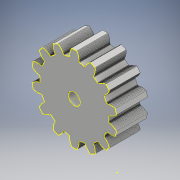
# Autodesk Inventor part: Engranaje_V_G
Saved by Autodesk Inventor 2017 (Build 210142000, 142)
## iProperties
Created: 2016-10-02
Part Number: Engranaje_V_G
Material: Generic
Document SubType Name: Modeling
Designer: CASA
Density: 1 g/cm^3
Appearance: Default
Author: CASA
Autodesk Inventor part; units mm, degrees
(part 1 of 2)
ref_plane "YZ Plane" through (0, 0, 0) normal (1, 0, 0) x (0, 1, 0)
ref_plane "XZ Plane" through (0, 0, 0) normal (0, 1, 0) x (-1, 0, 0)
ref_plane "XY Plane" through (0, 0, 0) normal (0, 0, 1) x (1, 0, 0)
sketch "Sketch4" plane through (0, 0, 0) normal (0, 1, 0) x (-1, 0, 0)
  line L0 (0.4842, 0.4117) -> (0.4817, 0.3929)
  line L1 (0.4817, 0.3929) -> (0.4745, 0.3754)
  line L2 (0.4745, 0.3754) -> (0.4629, 0.3604)
  line L3 (0.4629, 0.3604) -> (0.4479, 0.3489)
  line L4 (0.4479, 0.3489) -> (0.4304, 0.3416)
  line L5 (0.4304, 0.3416) -> (0.4117, 0.3392)
  line L6 (0.4117, 0.3392) -> (0.3929, 0.3416)
  line L7 (0.3929, 0.3416) -> (0.3754, 0.3489)
  line L8 (0.3754, 0.3489) -> (0.3604, 0.3604)
  line L9 (0.3604, 0.3604) -> (0.3489, 0.3754)
  line L10 (0.3489, 0.3754) -> (0.3416, 0.3929)
  line L11 (0.3416, 0.3929) -> (0.3392, 0.4117)
  line L12 (0.3392, 0.4117) -> (0.3416, 0.4304)
  line L13 (0.3416, 0.4304) -> (0.3489, 0.4479)
  line L14 (0.3489, 0.4479) -> (0.3604, 0.4629)
  line L15 (0.3604, 0.4629) -> (0.3754, 0.4745)
  line L16 (0.3754, 0.4745) -> (0.3929, 0.4817)
  line L17 (0.3929, 0.4817) -> (0.4117, 0.4842)
  line L18 (0.4117, 0.4842) -> (0.4304, 0.4817)
  line L19 (0.4304, 0.4817) -> (0.4479, 0.4745)
  line L20 (0.4479, 0.4745) -> (0.4629, 0.4629)
  line L21 (0.4629, 0.4629) -> (0.4745, 0.4479)
  line L22 (0.4745, 0.4479) -> (0.4817, 0.4304)
  line L23 (0.4817, 0.4304) -> (0.4842, 0.4117)
  line L24 (0.0797, 0.4378) -> (0.0785, 0.4393)
  line L25 (0.0785, 0.4393) -> (0.0772, 0.4404)
  line L26 (0.0772, 0.4404) -> (0.076, 0.4413)
  line L27 (0.076, 0.4413) -> (0.0747, 0.442)
  line L28 (0.0747, 0.442) -> (0.0734, 0.4426)
  line L29 (0.0734, 0.4426) -> (0.0708, 0.4437)
  line L30 (0.0708, 0.4437) -> (0.0682, 0.4445)
  line L31 (0.0682, 0.4445) -> (0.0656, 0.4451)
  line L32 (0.0656, 0.4451) -> (0.0604, 0.4462)
  line L33 (0.0604, 0.4462) -> (0.0552, 0.4478)
  line L34 (0.0552, 0.4478) -> (0.05, 0.4497)
  line L35 (0.05, 0.4497) -> (0.0449, 0.452)
  line L36 (0.0449, 0.452) -> (0.0398, 0.4545)
  line L37 (0.0398, 0.4545) -> (0.0348, 0.4573)
  line L38 (0.0348, 0.4573) -> (0.0298, 0.4603)
  line L39 (0.0298, 0.4603) -> (0.0248, 0.4636)
  line L40 (0.0248, 0.4636) -> (0.0199, 0.467)
  line L41 (0.0199, 0.467) -> (0.015, 0.4707)
  line L42 (0.015, 0.4707) -> (0.0102, 0.4745)
  line L43 (0.0102, 0.4745) -> (0.0055, 0.4786)
  line L44 (0.0055, 0.4786) -> (0.0167, 0.5276)
  line L45 (0.0167, 0.5276) -> (0.0227, 0.5292)
  line L46 (0.0227, 0.5292) -> (0.0287, 0.5306)
  line L47 (0.0287, 0.5306) -> (0.0347, 0.5318)
  line L48 (0.0347, 0.5318) -> (0.0406, 0.5328)
  line L49 (0.0406, 0.5328) -> (0.0465, 0.5335)
  line L50 (0.0465, 0.5335) -> (0.0523, 0.5341)
  line L51 (0.0523, 0.5341) -> (0.058, 0.5344)
  line L52 (0.058, 0.5344) -> (0.0637, 0.5345)
  line L53 (0.0637, 0.5345) -> (0.0693, 0.5343)
  line L54 (0.0693, 0.5343) -> (0.0748, 0.5338)
  line L55 (0.0748, 0.5338) -> (0.0802, 0.5329)
  line L56 (0.0802, 0.5329) -> (0.0854, 0.5316)
  line L57 (0.0854, 0.5316) -> (0.088, 0.5311)
  line L58 (0.088, 0.5311) -> (0.0907, 0.5307)
  line L59 (0.0907, 0.5307) -> (0.0935, 0.5305)
  line L60 (0.0935, 0.5305) -> (0.0949, 0.5305)
  line L61 (0.0949, 0.5305) -> (0.0964, 0.5307)
  line L62 (0.0964, 0.5307) -> (0.0979, 0.5309)
  line L63 (0.0979, 0.5309) -> (0.0995, 0.5313)
  line L64 (0.0995, 0.5313) -> (0.1012, 0.5322)
  line L65 (0.1012, 0.5322) -> (0.1038, 0.535)
  line L66 (0.1038, 0.535) -> (0.1233, 0.5755)
  line L67 (0.1233, 0.5755) -> (0.1239, 0.5792)
  line L68 (0.1239, 0.5792) -> (0.1235, 0.5811)
  line L69 (0.1235, 0.5811) -> (0.1228, 0.5826)
  line L70 (0.1228, 0.5826) -> (0.1221, 0.584)
  line L71 (0.1221, 0.584) -> (0.1212, 0.5852)
  line L72 (0.1212, 0.5852) -> (0.1204, 0.5863)
  line L73 (0.1204, 0.5863) -> (0.1185, 0.5884)
  line L74 (0.1185, 0.5884) -> (0.1165, 0.5903)
  line L75 (0.1165, 0.5903) -> (0.1144, 0.592)
  line L76 (0.1144, 0.592) -> (0.1102, 0.5952)
  line L77 (0.1102, 0.5952) -> (0.1061, 0.5989)
  line L78 (0.1061, 0.5989) -> (0.1023, 0.6029)
  line L79 (0.1023, 0.6029) -> (0.0987, 0.6071)
  line L80 (0.0987, 0.6071) -> (0.0952, 0.6116)
  line L81 (0.0952, 0.6116) -> (0.0919, 0.6163)
  line L82 (0.0919, 0.6163) -> (0.0887, 0.6212)
  line L83 (0.0887, 0.6212) -> (0.0856, 0.6263)
  line L84 (0.0856, 0.6263) -> (0.0827, 0.6315)
  line L85 (0.0827, 0.6315) -> (0.0799, 0.6369)
  line L86 (0.0799, 0.6369) -> (0.0773, 0.6425)
  line L87 (0.0773, 0.6425) -> (0.0747, 0.6482)
  line L88 (0.0747, 0.6482) -> (0.1061, 0.6875)
  line L89 (0.1061, 0.6875) -> (0.1122, 0.6863)
  line L90 (0.1122, 0.6863) -> (0.1182, 0.685)
  line L91 (0.1182, 0.685) -> (0.1241, 0.6835)
  line L92 (0.1241, 0.6835) -> (0.1299, 0.6818)
  line L93 (0.1299, 0.6818) -> (0.1355, 0.6799)
  line L94 (0.1355, 0.6799) -> (0.141, 0.6779)
  line L95 (0.141, 0.6779) -> (0.1463, 0.6757)
  line L96 (0.1463, 0.6757) -> (0.1515, 0.6733)
  line L97 (0.1515, 0.6733) -> (0.1564, 0.6707)
  line L98 (0.1564, 0.6707) -> (0.1612, 0.6679)
  line L99 (0.1612, 0.6679) -> (0.1656, 0.6648)
  line L100 (0.1656, 0.6648) -> (0.1697, 0.6613)
  line L101 (0.1697, 0.6613) -> (0.1719, 0.6597)
  line L102 (0.1719, 0.6597) -> (0.1741, 0.6582)
  line L103 (0.1741, 0.6582) -> (0.1766, 0.6568)
  line L104 (0.1766, 0.6568) -> (0.1779, 0.6562)
  line L105 (0.1779, 0.6562) -> (0.1792, 0.6557)
  line L106 (0.1792, 0.6557) -> (0.1807, 0.6552)
  line L107 (0.1807, 0.6552) -> (0.1823, 0.6549)
  line L108 (0.1823, 0.6549) -> (0.1843, 0.6549)
  line L109 (0.1843, 0.6549) -> (0.1878, 0.6564)
  line L110 (0.1878, 0.6564) -> (0.2229, 0.6844)
  line L111 (0.2229, 0.6844) -> (0.2251, 0.6875)
  line L112 (0.2251, 0.6875) -> (0.2255, 0.6894)
  line L113 (0.2255, 0.6894) -> (0.2256, 0.691)
  line L114 (0.2256, 0.691) -> (0.2255, 0.6926)
  line L115 (0.2255, 0.6926) -> (0.2253, 0.694)
  line L116 (0.2253, 0.694) -> (0.225, 0.6954)
  line L117 (0.225, 0.6954) -> (0.2242, 0.6981)
  line L118 (0.2242, 0.6981) -> (0.2232, 0.7006)
  line L119 (0.2232, 0.7006) -> (0.2221, 0.7031)
  line L120 (0.2221, 0.7031) -> (0.2197, 0.7079)
  line L121 (0.2197, 0.7079) -> (0.2176, 0.7129)
  line L122 (0.2176, 0.7129) -> (0.2159, 0.7181)
  line L123 (0.2159, 0.7181) -> (0.2145, 0.7236)
  line L124 (0.2145, 0.7236) -> (0.2133, 0.7291)
  line L125 (0.2133, 0.7291) -> (0.2123, 0.7348)
  line L126 (0.2123, 0.7348) -> (0.2116, 0.7406)
  line L127 (0.2116, 0.7406) -> (0.211, 0.7465)
  line L128 (0.211, 0.7465) -> (0.2107, 0.7525)
  line L129 (0.2107, 0.7525) -> (0.2105, 0.7585)
  line L130 (0.2105, 0.7585) -> (0.2105, 0.7647)
  line L131 (0.2105, 0.7647) -> (0.2107, 0.771)
  line L132 (0.2107, 0.771) -> (0.256, 0.7928)
  line L133 (0.256, 0.7928) -> (0.261, 0.789)
  line L134 (0.261, 0.789) -> (0.2659, 0.7852)
  line L135 (0.2659, 0.7852) -> (0.2705, 0.7813)
  line L136 (0.2705, 0.7813) -> (0.275, 0.7773)
  line L137 (0.275, 0.7773) -> (0.2793, 0.7732)
  line L138 (0.2793, 0.7732) -> (0.2833, 0.769)
  line L139 (0.2833, 0.769) -> (0.2872, 0.7647)
  line L140 (0.2872, 0.7647) -> (0.2908, 0.7603)
  line L141 (0.2908, 0.7603) -> (0.2941, 0.7558)
  line L142 (0.2941, 0.7558) -> (0.2971, 0.7512)
  line L143 (0.2971, 0.7512) -> (0.2998, 0.7465)
  line L144 (0.2998, 0.7465) -> (0.302, 0.7416)
  line L145 (0.302, 0.7416) -> (0.3032, 0.7392)
  line L146 (0.3032, 0.7392) -> (0.3046, 0.7368)
  line L147 (0.3046, 0.7368) -> (0.3062, 0.7345)
  line L148 (0.3062, 0.7345) -> (0.3071, 0.7334)
  line L149 (0.3071, 0.7334) -> (0.3081, 0.7323)
  line L150 (0.3081, 0.7323) -> (0.3093, 0.7313)
  line L151 (0.3093, 0.7313) -> (0.3106, 0.7303)
  line L152 (0.3106, 0.7303) -> (0.3123, 0.7295)
  line L153 (0.3123, 0.7295) -> (0.3161, 0.7293)
  line L154 (0.3161, 0.7293) -> (0.3599, 0.7393)
  line L155 (0.3599, 0.7393) -> (0.3633, 0.7411)
  line L156 (0.3633, 0.7411) -> (0.3644, 0.7426)
  line L157 (0.3644, 0.7426) -> (0.3652, 0.7441)
  line L158 (0.3652, 0.7441) -> (0.3658, 0.7455)
  line L159 (0.3658, 0.7455) -> (0.3663, 0.7469)
  line L160 (0.3663, 0.7469) -> (0.3666, 0.7483)
  line L161 (0.3666, 0.7483) -> (0.3671, 0.7511)
  line L162 (0.3671, 0.7511) -> (0.3673, 0.7538)
  line L163 (0.3673, 0.7538) -> (0.3673, 0.7565)
  line L164 (0.3673, 0.7565) -> (0.3672, 0.7618)
  line L165 (0.3672, 0.7618) -> (0.3676, 0.7673)
  line L166 (0.3676, 0.7673) -> (0.3683, 0.7727)
  line L167 (0.3683, 0.7727) -> (0.3694, 0.7782)
  line L168 (0.3694, 0.7782) -> (0.3707, 0.7837)
  line L169 (0.3707, 0.7837) -> (0.3723, 0.7893)
  line L170 (0.3723, 0.7893) -> (0.3741, 0.7948)
  line L171 (0.3741, 0.7948) -> (0.3762, 0.8004)
  line L172 (0.3762, 0.8004) -> (0.3784, 0.8059)
  line L173 (0.3784, 0.8059) -> (0.3809, 0.8115)
  line L174 (0.3809, 0.8115) -> (0.3836, 0.817)
  line L175 (0.3836, 0.817) -> (0.3865, 0.8226)
  line L176 (0.3865, 0.8226) -> (0.4368, 0.8226)
  line L177 (0.4368, 0.8226) -> (0.4397, 0.817)
  line L178 (0.4397, 0.817) -> (0.4424, 0.8115)
  line L179 (0.4424, 0.8115) -> (0.4449, 0.8059)
  line L180 (0.4449, 0.8059) -> (0.4472, 0.8004)
  line L181 (0.4472, 0.8004) -> (0.4492, 0.7948)
  line L182 (0.4492, 0.7948) -> (0.4511, 0.7893)
  line L183 (0.4511, 0.7893) -> (0.4527, 0.7837)
  line L184 (0.4527, 0.7837) -> (0.454, 0.7782)
  line L185 (0.454, 0.7782) -> (0.455, 0.7727)
  line L186 (0.455, 0.7727) -> (0.4558, 0.7673)
  line L187 (0.4558, 0.7673) -> (0.4561, 0.7618)
  line L188 (0.4561, 0.7618) -> (0.456, 0.7565)
  line L189 (0.456, 0.7565) -> (0.4561, 0.7538)
  line L190 (0.4561, 0.7538) -> (0.4563, 0.7511)
  line L191 (0.4563, 0.7511) -> (0.4567, 0.7483)
  line L192 (0.4567, 0.7483) -> (0.4571, 0.7469)
  line L193 (0.4571, 0.7469) -> (0.4575, 0.7455)
  line L194 (0.4575, 0.7455) -> (0.4581, 0.7441)
  line L195 (0.4581, 0.7441) -> (0.4589, 0.7426)
  line L196 (0.4589, 0.7426) -> (0.4601, 0.7411)
  line L197 (0.4601, 0.7411) -> (0.4634, 0.7393)
  line L198 (0.4634, 0.7393) -> (0.5072, 0.7293)
  line L199 (0.5072, 0.7293) -> (0.511, 0.7295)
  line L200 (0.511, 0.7295) -> (0.5127, 0.7303)
  line L201 (0.5127, 0.7303) -> (0.5141, 0.7313)
  line L202 (0.5141, 0.7313) -> (0.5152, 0.7323)
  line L203 (0.5152, 0.7323) -> (0.5162, 0.7334)
  line L204 (0.5162, 0.7334) -> (0.5171, 0.7345)
  line L205 (0.5171, 0.7345) -> (0.5187, 0.7368)
  line L206 (0.5187, 0.7368) -> (0.5201, 0.7392)
  line L207 (0.5201, 0.7392) -> (0.5213, 0.7416)
  line L208 (0.5213, 0.7416) -> (0.5235, 0.7465)
  line L209 (0.5235, 0.7465) -> (0.5262, 0.7512)
  line L210 (0.5262, 0.7512) -> (0.5293, 0.7558)
  line L211 (0.5293, 0.7558) -> (0.5326, 0.7603)
  line L212 (0.5326, 0.7603) -> (0.5362, 0.7647)
  line L213 (0.5362, 0.7647) -> (0.54, 0.769)
  line L214 (0.54, 0.769) -> (0.5441, 0.7732)
  line L215 (0.5441, 0.7732) -> (0.5483, 0.7773)
  line L216 (0.5483, 0.7773) -> (0.5528, 0.7813)
  line L217 (0.5528, 0.7813) -> (0.5575, 0.7852)
  line L218 (0.5575, 0.7852) -> (0.5623, 0.789)
  line L219 (0.5623, 0.789) -> (0.5673, 0.7928)
  line L220 (0.5673, 0.7928) -> (0.6126, 0.771)
  line L221 (0.6126, 0.771) -> (0.6128, 0.7647)
  line L222 (0.6128, 0.7647) -> (0.6128, 0.7585)
  line L223 (0.6128, 0.7585) -> (0.6127, 0.7525)
  line L224 (0.6127, 0.7525) -> (0.6123, 0.7465)
  line L225 (0.6123, 0.7465) -> (0.6118, 0.7406)
  line L226 (0.6118, 0.7406) -> (0.611, 0.7348)
  line L227 (0.611, 0.7348) -> (0.61, 0.7291)
  line L228 (0.61, 0.7291) -> (0.6088, 0.7236)
  line L229 (0.6088, 0.7236) -> (0.6074, 0.7181)
  line L230 (0.6074, 0.7181) -> (0.6057, 0.7129)
  line L231 (0.6057, 0.7129) -> (0.6037, 0.7079)
  line L232 (0.6037, 0.7079) -> (0.6013, 0.7031)
  line L233 (0.6013, 0.7031) -> (0.6001, 0.7006)
  line L234 (0.6001, 0.7006) -> (0.5991, 0.6981)
  line L235 (0.5991, 0.6981) -> (0.5983, 0.6954)
  line L236 (0.5983, 0.6954) -> (0.598, 0.694)
  line L237 (0.598, 0.694) -> (0.5978, 0.6926)
  line L238 (0.5978, 0.6926) -> (0.5977, 0.691)
  line L239 (0.5977, 0.691) -> (0.5978, 0.6894)
  line L240 (0.5978, 0.6894) -> (0.5982, 0.6875)
  line L241 (0.5982, 0.6875) -> (0.6004, 0.6844)
  line L242 (0.6004, 0.6844) -> (0.6356, 0.6564)
  line L243 (0.6356, 0.6564) -> (0.6391, 0.6549)
  line L244 (0.6391, 0.6549) -> (0.641, 0.6549)
  line L245 (0.641, 0.6549) -> (0.6426, 0.6552)
  line L246 (0.6426, 0.6552) -> (0.6441, 0.6557)
  line L247 (0.6441, 0.6557) -> (0.6455, 0.6562)
  line L248 (0.6455, 0.6562) -> (0.6468, 0.6568)
  line L249 (0.6468, 0.6568) -> (0.6492, 0.6582)
  line L250 (0.6492, 0.6582) -> (0.6515, 0.6597)
  line L251 (0.6515, 0.6597) -> (0.6536, 0.6613)
  line L252 (0.6536, 0.6613) -> (0.6577, 0.6648)
  line L253 (0.6577, 0.6648) -> (0.6622, 0.6679)
  line L254 (0.6622, 0.6679) -> (0.6669, 0.6707)
  line L255 (0.6669, 0.6707) -> (0.6719, 0.6733)
  line L256 (0.6719, 0.6733) -> (0.677, 0.6757)
  line L257 (0.677, 0.6757) -> (0.6823, 0.6779)
  line L258 (0.6823, 0.6779) -> (0.6878, 0.6799)
  line L259 (0.6878, 0.6799) -> (0.6935, 0.6818)
  line L260 (0.6935, 0.6818) -> (0.6992, 0.6835)
  line L261 (0.6992, 0.6835) -> (0.7051, 0.685)
  line L262 (0.7051, 0.685) -> (0.7111, 0.6863)
  line L263 (0.7111, 0.6863) -> (0.7173, 0.6875)
  line L264 (0.7173, 0.6875) -> (0.7486, 0.6482)
  line L265 (0.7486, 0.6482) -> (0.7461, 0.6425)
  line L266 (0.7461, 0.6425) -> (0.7434, 0.6369)
  line L267 (0.7434, 0.6369) -> (0.7406, 0.6315)
  line L268 (0.7406, 0.6315) -> (0.7377, 0.6263)
  line L269 (0.7377, 0.6263) -> (0.7347, 0.6212)
  line L270 (0.7347, 0.6212) -> (0.7315, 0.6163)
  line L271 (0.7315, 0.6163) -> (0.7281, 0.6116)
  line L272 (0.7281, 0.6116) -> (0.7247, 0.6071)
  line L273 (0.7247, 0.6071) -> (0.721, 0.6029)
  line L274 (0.721, 0.6029) -> (0.7172, 0.5989)
  line L275 (0.7172, 0.5989) -> (0.7132, 0.5952)
  line L276 (0.7132, 0.5952) -> (0.7089, 0.592)
  line L277 (0.7089, 0.592) -> (0.7068, 0.5903)
  line L278 (0.7068, 0.5903) -> (0.7049, 0.5884)
  line L279 (0.7049, 0.5884) -> (0.703, 0.5863)
  line L280 (0.703, 0.5863) -> (0.7021, 0.5852)
  line L281 (0.7021, 0.5852) -> (0.7013, 0.584)
  line L282 (0.7013, 0.584) -> (0.7005, 0.5826)
  line L283 (0.7005, 0.5826) -> (0.6999, 0.5811)
  line L284 (0.6999, 0.5811) -> (0.6994, 0.5792)
  line L285 (0.6994, 0.5792) -> (0.7001, 0.5755)
  line L286 (0.7001, 0.5755) -> (0.7196, 0.535)
  line L287 (0.7196, 0.535) -> (0.7221, 0.5322)
  line L288 (0.7221, 0.5322) -> (0.7238, 0.5314)
  line L289 (0.7238, 0.5314) -> (0.7254, 0.5309)
  line L290 (0.7254, 0.5309) -> (0.727, 0.5307)
  line L291 (0.727, 0.5307) -> (0.7284, 0.5305)
  line L292 (0.7284, 0.5305) -> (0.7299, 0.5305)
  line L293 (0.7299, 0.5305) -> (0.7326, 0.5307)
  line L294 (0.7326, 0.5307) -> (0.7353, 0.5311)
  line L295 (0.7353, 0.5311) -> (0.738, 0.5316)
  line L296 (0.738, 0.5316) -> (0.7432, 0.5329)
  line L297 (0.7432, 0.5329) -> (0.7485, 0.5338)
  line L298 (0.7485, 0.5338) -> (0.754, 0.5343)
  line L299 (0.754, 0.5343) -> (0.7596, 0.5345)
  line L300 (0.7596, 0.5345) -> (0.7653, 0.5344)
  line L301 (0.7653, 0.5344) -> (0.7711, 0.5341)
  line L302 (0.7711, 0.5341) -> (0.7769, 0.5336)
  line L303 (0.7769, 0.5336) -> (0.7827, 0.5328)
  line L304 (0.7827, 0.5328) -> (0.7887, 0.5318)
  line L305 (0.7887, 0.5318) -> (0.7946, 0.5306)
  line L306 (0.7946, 0.5306) -> (0.8006, 0.5292)
  line L307 (0.8006, 0.5292) -> (0.8067, 0.5276)
  line L308 (0.8067, 0.5276) -> (0.8179, 0.4786)
  line L309 (0.8179, 0.4786) -> (0.8131, 0.4745)
  line L310 (0.8131, 0.4745) -> (0.8083, 0.4707)
  line L311 (0.8083, 0.4707) -> (0.8034, 0.467)
  line L312 (0.8034, 0.467) -> (0.7985, 0.4635)
  line L313 (0.7985, 0.4635) -> (0.7935, 0.4603)
  line L314 (0.7935, 0.4603) -> (0.7885, 0.4573)
  line L315 (0.7885, 0.4573) -> (0.7835, 0.4545)
  line L316 (0.7835, 0.4545) -> (0.7784, 0.452)
  line L317 (0.7784, 0.452) -> (0.7733, 0.4497)
  line L318 (0.7733, 0.4497) -> (0.7681, 0.4478)
  line L319 (0.7681, 0.4478) -> (0.7629, 0.4463)
  line L320 (0.7629, 0.4463) -> (0.7577, 0.4452)
  line L321 (0.7577, 0.4452) -> (0.7551, 0.4445)
  line L322 (0.7551, 0.4445) -> (0.7525, 0.4437)
  line L323 (0.7525, 0.4437) -> (0.7499, 0.4427)
  line L324 (0.7499, 0.4427) -> (0.7486, 0.442)
  line L325 (0.7486, 0.442) -> (0.7473, 0.4413)
  line L326 (0.7473, 0.4413) -> (0.7461, 0.4404)
  line L327 (0.7461, 0.4404) -> (0.7448, 0.4393)
  line L328 (0.7448, 0.4393) -> (0.7436, 0.4378)
  line L329 (0.7436, 0.4378) -> (0.7425, 0.4342)
  line L330 (0.7425, 0.4342) -> (0.7425, 0.3892)
  line L331 (0.7425, 0.3892) -> (0.7436, 0.3856)
  line L332 (0.7436, 0.3856) -> (0.7448, 0.3841)
  line L333 (0.7448, 0.3841) -> (0.7461, 0.383)
  line L334 (0.7461, 0.383) -> (0.7473, 0.3821)
  line L335 (0.7473, 0.3821) -> (0.7486, 0.3813)
  line L336 (0.7486, 0.3813) -> (0.7499, 0.3807)
  line L337 (0.7499, 0.3807) -> (0.7525, 0.3797)
  line L338 (0.7525, 0.3797) -> (0.7551, 0.3788)
  line L339 (0.7551, 0.3788) -> (0.7577, 0.3782)
  line L340 (0.7577, 0.3782) -> (0.7629, 0.3771)
  line L341 (0.7629, 0.3771) -> (0.7681, 0.3756)
  line L342 (0.7681, 0.3756) -> (0.7733, 0.3736)
  line L343 (0.7733, 0.3736) -> (0.7784, 0.3714)
  line L344 (0.7784, 0.3714) -> (0.7835, 0.3688)
  line L345 (0.7835, 0.3688) -> (0.7885, 0.3661)
  line L346 (0.7885, 0.3661) -> (0.7935, 0.363)
  line L347 (0.7935, 0.363) -> (0.7985, 0.3598)
  line L348 (0.7985, 0.3598) -> (0.8034, 0.3563)
  line L349 (0.8034, 0.3563) -> (0.8083, 0.3527)
  line L350 (0.8083, 0.3527) -> (0.8131, 0.3488)
  line L351 (0.8131, 0.3488) -> (0.8179, 0.3447)
  line L352 (0.8179, 0.3447) -> (0.8067, 0.2957)
  line L353 (0.8067, 0.2957) -> (0.8006, 0.2941)
  line L354 (0.8006, 0.2941) -> (0.7946, 0.2927)
  line L355 (0.7946, 0.2927) -> (0.7887, 0.2915)
  line L356 (0.7887, 0.2915) -> (0.7827, 0.2906)
  line L357 (0.7827, 0.2906) -> (0.7769, 0.2898)
  line L358 (0.7769, 0.2898) -> (0.7711, 0.2892)
  line L359 (0.7711, 0.2892) -> (0.7653, 0.2889)
  line L360 (0.7653, 0.2889) -> (0.7596, 0.2888)
  line L361 (0.7596, 0.2888) -> (0.754, 0.289)
  line L362 (0.754, 0.289) -> (0.7485, 0.2895)
  line L363 (0.7485, 0.2895) -> (0.7432, 0.2904)
  line L364 (0.7432, 0.2904) -> (0.738, 0.2917)
  line L365 (0.738, 0.2917) -> (0.7353, 0.2923)
  line L366 (0.7353, 0.2923) -> (0.7326, 0.2927)
  line L367 (0.7326, 0.2927) -> (0.7299, 0.2928)
  line L368 (0.7299, 0.2928) -> (0.7284, 0.2928)
  line L369 (0.7284, 0.2928) -> (0.727, 0.2927)
  line L370 (0.727, 0.2927) -> (0.7254, 0.2924)
  line L371 (0.7254, 0.2924) -> (0.7238, 0.292)
  line L372 (0.7238, 0.292) -> (0.7221, 0.2912)
  line L373 (0.7221, 0.2912) -> (0.7196, 0.2883)
  line L374 (0.7196, 0.2883) -> (0.7001, 0.2479)
  line L375 (0.7001, 0.2479) -> (0.6994, 0.2441)
  line L376 (0.6994, 0.2441) -> (0.6999, 0.2422)
  line L377 (0.6999, 0.2422) -> (0.7005, 0.2407)
  line L378 (0.7005, 0.2407) -> (0.7013, 0.2394)
  line L379 (0.7013, 0.2394) -> (0.7021, 0.2381)
  line L380 (0.7021, 0.2381) -> (0.703, 0.237)
  line L381 (0.703, 0.237) -> (0.7049, 0.2349)
  line L382 (0.7049, 0.2349) -> (0.7068, 0.2331)
  line L383 (0.7068, 0.2331) -> (0.7089, 0.2314)
  line L384 (0.7089, 0.2314) -> (0.7132, 0.2281)
  line L385 (0.7132, 0.2281) -> (0.7172, 0.2244)
  line L386 (0.7172, 0.2244) -> (0.721, 0.2205)
  line L387 (0.721, 0.2205) -> (0.7247, 0.2162)
  line L388 (0.7247, 0.2162) -> (0.7281, 0.2117)
  line L389 (0.7281, 0.2117) -> (0.7315, 0.207)
  line L390 (0.7315, 0.207) -> (0.7347, 0.2021)
  line L391 (0.7347, 0.2021) -> (0.7377, 0.1971)
  line L392 (0.7377, 0.1971) -> (0.7406, 0.1918)
  line L393 (0.7406, 0.1918) -> (0.7434, 0.1864)
  line L394 (0.7434, 0.1864) -> (0.7461, 0.1809)
  line L395 (0.7461, 0.1809) -> (0.7486, 0.1751)
  line L396 (0.7486, 0.1751) -> (0.7173, 0.1358)
  line L397 (0.7173, 0.1358) -> (0.7111, 0.137)
  line L398 (0.7111, 0.137) -> (0.7051, 0.1384)
  line L399 (0.7051, 0.1384) -> (0.6992, 0.1399)
  line L400 (0.6992, 0.1399) -> (0.6935, 0.1416)
  line L401 (0.6935, 0.1416) -> (0.6878, 0.1434)
  line L402 (0.6878, 0.1434) -> (0.6823, 0.1454)
  line L403 (0.6823, 0.1454) -> (0.677, 0.1476)
  line L404 (0.677, 0.1476) -> (0.6719, 0.15)
  line L405 (0.6719, 0.15) -> (0.6669, 0.1526)
  line L406 (0.6669, 0.1526) -> (0.6622, 0.1555)
  line L407 (0.6622, 0.1555) -> (0.6577, 0.1586)
  line L408 (0.6577, 0.1586) -> (0.6536, 0.162)
  line L409 (0.6536, 0.162) -> (0.6515, 0.1637)
  line L410 (0.6515, 0.1637) -> (0.6492, 0.1652)
  line L411 (0.6492, 0.1652) -> (0.6468, 0.1665)
  line L412 (0.6468, 0.1665) -> (0.6455, 0.1671)
  line L413 (0.6455, 0.1671) -> (0.6441, 0.1677)
  line L414 (0.6441, 0.1677) -> (0.6426, 0.1681)
  line L415 (0.6426, 0.1681) -> (0.641, 0.1684)
  line L416 (0.641, 0.1684) -> (0.6391, 0.1684)
  line L417 (0.6391, 0.1684) -> (0.6356, 0.167)
  line L418 (0.6356, 0.167) -> (0.6004, 0.139)
  line L419 (0.6004, 0.139) -> (0.5982, 0.1358)
  line L420 (0.5982, 0.1358) -> (0.5978, 0.134)
  line L421 (0.5978, 0.134) -> (0.5977, 0.1323)
  line L422 (0.5977, 0.1323) -> (0.5978, 0.1308)
  line L423 (0.5978, 0.1308) -> (0.598, 0.1293)
  line L424 (0.598, 0.1293) -> (0.5983, 0.1279)
  line L425 (0.5983, 0.1279) -> (0.5991, 0.1252)
  line L426 (0.5991, 0.1252) -> (0.6001, 0.1227)
  line L427 (0.6001, 0.1227) -> (0.6013, 0.1203)
  line L428 (0.6013, 0.1203) -> (0.6037, 0.1155)
  line L429 (0.6037, 0.1155) -> (0.6057, 0.1104)
  line L430 (0.6057, 0.1104) -> (0.6074, 0.1052)
  line L431 (0.6074, 0.1052) -> (0.6088, 0.0998)
  line L432 (0.6088, 0.0998) -> (0.61, 0.0942)
  line L433 (0.61, 0.0942) -> (0.611, 0.0885)
  line L434 (0.611, 0.0885) -> (0.6118, 0.0828)
  line L435 (0.6118, 0.0828) -> (0.6123, 0.0769)
  line L436 (0.6123, 0.0769) -> (0.6127, 0.0709)
  line L437 (0.6127, 0.0709) -> (0.6128, 0.0648)
  line L438 (0.6128, 0.0648) -> (0.6128, 0.0586)
  line L439 (0.6128, 0.0586) -> (0.6126, 0.0524)
  line L440 (0.6126, 0.0524) -> (0.5673, 0.0306)
  line L441 (0.5673, 0.0306) -> (0.5623, 0.0343)
  line L442 (0.5623, 0.0343) -> (0.5575, 0.0381)
  line L443 (0.5575, 0.0381) -> (0.5528, 0.042)
  line L444 (0.5528, 0.042) -> (0.5483, 0.046)
  line L445 (0.5483, 0.046) -> (0.5441, 0.0502)
  line L446 (0.5441, 0.0502) -> (0.54, 0.0544)
  line L447 (0.54, 0.0544) -> (0.5362, 0.0587)
  line L448 (0.5362, 0.0587) -> (0.5326, 0.0631)
  line L449 (0.5326, 0.0631) -> (0.5293, 0.0675)
  line L450 (0.5293, 0.0675) -> (0.5262, 0.0721)
  line L451 (0.5262, 0.0721) -> (0.5235, 0.0769)
  line L452 (0.5235, 0.0769) -> (0.5213, 0.0818)
  line L453 (0.5213, 0.0818) -> (0.5201, 0.0842)
  line L454 (0.5201, 0.0842) -> (0.5187, 0.0865)
  line L455 (0.5187, 0.0865) -> (0.5171, 0.0888)
  line L456 (0.5171, 0.0888) -> (0.5162, 0.0899)
  line L457 (0.5162, 0.0899) -> (0.5152, 0.091)
  line L458 (0.5152, 0.091) -> (0.5141, 0.092)
  line L459 (0.5141, 0.092) -> (0.5127, 0.093)
  line L460 (0.5127, 0.093) -> (0.511, 0.0938)
  line L461 (0.511, 0.0938) -> (0.5072, 0.0941)
  line L462 (0.5072, 0.0941) -> (0.4634, 0.0841)
  line L463 (0.4634, 0.0841) -> (0.4601, 0.0822)
  line L464 (0.4601, 0.0822) -> (0.4589, 0.0807)
  line L465 (0.4589, 0.0807) -> (0.4581, 0.0792)
  line L466 (0.4581, 0.0792) -> (0.4575, 0.0778)
  line L467 (0.4575, 0.0778) -> (0.4571, 0.0764)
  line L468 (0.4571, 0.0764) -> (0.4567, 0.075)
  line L469 (0.4567, 0.075) -> (0.4563, 0.0723)
  line L470 (0.4563, 0.0723) -> (0.4561, 0.0695)
  line L471 (0.4561, 0.0695) -> (0.456, 0.0669)
  line L472 (0.456, 0.0669) -> (0.4561, 0.0615)
  line L473 (0.4561, 0.0615) -> (0.4558, 0.0561)
  line L474 (0.4558, 0.0561) -> (0.455, 0.0506)
  line L475 (0.455, 0.0506) -> (0.454, 0.0451)
  line L476 (0.454, 0.0451) -> (0.4527, 0.0396)
  line L477 (0.4527, 0.0396) -> (0.4511, 0.0341)
  line L478 (0.4511, 0.0341) -> (0.4492, 0.0285)
  line L479 (0.4492, 0.0285) -> (0.4472, 0.023)
  line L480 (0.4472, 0.023) -> (0.4449, 0.0174)
  line L481 (0.4449, 0.0174) -> (0.4424, 0.0119)
  line L482 (0.4424, 0.0119) -> (0.4397, 0.0063)
  line L483 (0.4397, 0.0063) -> (0.4368, 0.0008)
  line L484 (0.4368, 0.0008) -> (0.3865, 0.0008)
  line L485 (0.3865, 0.0008) -> (0.3836, 0.0063)
  line L486 (0.3836, 0.0063) -> (0.3809, 0.0119)
  line L487 (0.3809, 0.0119) -> (0.3784, 0.0174)
  line L488 (0.3784, 0.0174) -> (0.3762, 0.023)
  line L489 (0.3762, 0.023) -> (0.3741, 0.0285)
  line L490 (0.3741, 0.0285) -> (0.3723, 0.0341)
  line L491 (0.3723, 0.0341) -> (0.3707, 0.0396)
  line L492 (0.3707, 0.0396) -> (0.3694, 0.0451)
  line L493 (0.3694, 0.0451) -> (0.3683, 0.0506)
  line L494 (0.3683, 0.0506) -> (0.3676, 0.0561)
  line L495 (0.3676, 0.0561) -> (0.3672, 0.0615)
  line L496 (0.3672, 0.0615) -> (0.3673, 0.0669)
  line L497 (0.3673, 0.0669) -> (0.3673, 0.0695)
  line L498 (0.3673, 0.0695) -> (0.3671, 0.0723)
  line L499 (0.3671, 0.0723) -> (0.3666, 0.075)
  line L500 (0.3666, 0.075) -> (0.3663, 0.0764)
  line L501 (0.3663, 0.0764) -> (0.3658, 0.0778)
  line L502 (0.3658, 0.0778) -> (0.3652, 0.0792)
  line L503 (0.3652, 0.0792) -> (0.3644, 0.0807)
  line L504 (0.3644, 0.0807) -> (0.3633, 0.0822)
  line L505 (0.3633, 0.0822) -> (0.3599, 0.0841)
  line L506 (0.3599, 0.0841) -> (0.3161, 0.0941)
  line L507 (0.3161, 0.0941) -> (0.3123, 0.0938)
  line L508 (0.3123, 0.0938) -> (0.3106, 0.093)
  line L509 (0.3106, 0.093) -> (0.3093, 0.092)
  line L510 (0.3093, 0.092) -> (0.3081, 0.091)
  line L511 (0.3081, 0.091) -> (0.3071, 0.0899)
  line L512 (0.3071, 0.0899) -> (0.3062, 0.0888)
  line L513 (0.3062, 0.0888) -> (0.3046, 0.0865)
  line L514 (0.3046, 0.0865) -> (0.3032, 0.0842)
  line L515 (0.3032, 0.0842) -> (0.302, 0.0818)
  line L516 (0.302, 0.0818) -> (0.2998, 0.0769)
  line L517 (0.2998, 0.0769) -> (0.2971, 0.0721)
  line L518 (0.2971, 0.0721) -> (0.2941, 0.0675)
  line L519 (0.2941, 0.0675) -> (0.2908, 0.0631)
  line L520 (0.2908, 0.0631) -> (0.2872, 0.0587)
  line L521 (0.2872, 0.0587) -> (0.2833, 0.0544)
  line L522 (0.2833, 0.0544) -> (0.2793, 0.0502)
  line L523 (0.2793, 0.0502) -> (0.275, 0.046)
  line L524 (0.275, 0.046) -> (0.2705, 0.042)
  line L525 (0.2705, 0.042) -> (0.2659, 0.0381)
  line L526 (0.2659, 0.0381) -> (0.261, 0.0343)
  line L527 (0.261, 0.0343) -> (0.256, 0.0306)
  line L528 (0.256, 0.0306) -> (0.2107, 0.0524)
  line L529 (0.2107, 0.0524) -> (0.2105, 0.0586)
  line L530 (0.2105, 0.0586) -> (0.2105, 0.0648)
  line L531 (0.2105, 0.0648) -> (0.2107, 0.0709)
  line L532 (0.2107, 0.0709) -> (0.211, 0.0769)
  line L533 (0.211, 0.0769) -> (0.2116, 0.0828)
  line L534 (0.2116, 0.0828) -> (0.2123, 0.0885)
  line L535 (0.2123, 0.0885) -> (0.2133, 0.0942)
  line L536 (0.2133, 0.0942) -> (0.2145, 0.0998)
  line L537 (0.2145, 0.0998) -> (0.2159, 0.1052)
  line L538 (0.2159, 0.1052) -> (0.2176, 0.1104)
  line L539 (0.2176, 0.1104) -> (0.2197, 0.1155)
  line L540 (0.2197, 0.1155) -> (0.2221, 0.1203)
  line L541 (0.2221, 0.1203) -> (0.2232, 0.1227)
  line L542 (0.2232, 0.1227) -> (0.2242, 0.1252)
  line L543 (0.2242, 0.1252) -> (0.225, 0.1279)
  line L544 (0.225, 0.1279) -> (0.2253, 0.1293)
  line L545 (0.2253, 0.1293) -> (0.2255, 0.1308)
  line L546 (0.2255, 0.1308) -> (0.2256, 0.1323)
  line L547 (0.2256, 0.1323) -> (0.2255, 0.134)
  line L548 (0.2255, 0.134) -> (0.2251, 0.1358)
  line L549 (0.2251, 0.1358) -> (0.2229, 0.139)
  line L550 (0.2229, 0.139) -> (0.1878, 0.167)
  line L551 (0.1878, 0.167) -> (0.1843, 0.1684)
  line L552 (0.1843, 0.1684) -> (0.1823, 0.1684)
  line L553 (0.1823, 0.1684) -> (0.1807, 0.1681)
  line L554 (0.1807, 0.1681) -> (0.1792, 0.1677)
  line L555 (0.1792, 0.1677) -> (0.1779, 0.1671)
  line L556 (0.1779, 0.1671) -> (0.1766, 0.1665)
  line L557 (0.1766, 0.1665) -> (0.1741, 0.1652)
  line L558 (0.1741, 0.1652) -> (0.1719, 0.1637)
  line L559 (0.1719, 0.1637) -> (0.1697, 0.162)
  line L560 (0.1697, 0.162) -> (0.1656, 0.1586)
  line L561 (0.1656, 0.1586) -> (0.1612, 0.1555)
  line L562 (0.1612, 0.1555) -> (0.1564, 0.1526)
  line L563 (0.1564, 0.1526) -> (0.1515, 0.15)
  line L564 (0.1515, 0.15) -> (0.1463, 0.1476)
  line L565 (0.1463, 0.1476) -> (0.141, 0.1454)
  line L566 (0.141, 0.1454) -> (0.1355, 0.1434)
  line L567 (0.1355, 0.1434) -> (0.1299, 0.1416)
  line L568 (0.1299, 0.1416) -> (0.1241, 0.1399)
  line L569 (0.1241, 0.1399) -> (0.1182, 0.1384)
  line L570 (0.1182, 0.1384) -> (0.1122, 0.137)
  line L571 (0.1122, 0.137) -> (0.1061, 0.1358)
  line L572 (0.1061, 0.1358) -> (0.0747, 0.1751)
  line L573 (0.0747, 0.1751) -> (0.0773, 0.1809)
  line L574 (0.0773, 0.1809) -> (0.0799, 0.1864)
  line L575 (0.0799, 0.1864) -> (0.0827, 0.1918)
  line L576 (0.0827, 0.1918) -> (0.0856, 0.1971)
  line L577 (0.0856, 0.1971) -> (0.0887, 0.2021)
  line L578 (0.0887, 0.2021) -> (0.0919, 0.207)
  line L579 (0.0919, 0.207) -> (0.0952, 0.2117)
  line L580 (0.0952, 0.2117) -> (0.0987, 0.2162)
  line L581 (0.0987, 0.2162) -> (0.1023, 0.2205)
  line L582 (0.1023, 0.2205) -> (0.1061, 0.2244)
  line L583 (0.1061, 0.2244) -> (0.1102, 0.2281)
  line L584 (0.1102, 0.2281) -> (0.1144, 0.2314)
  line L585 (0.1144, 0.2314) -> (0.1165, 0.2331)
  line L586 (0.1165, 0.2331) -> (0.1185, 0.2349)
  line L587 (0.1185, 0.2349) -> (0.1204, 0.237)
  line L588 (0.1204, 0.237) -> (0.1212, 0.2381)
  line L589 (0.1212, 0.2381) -> (0.1221, 0.2394)
  line L590 (0.1221, 0.2394) -> (0.1228, 0.2407)
  line L591 (0.1228, 0.2407) -> (0.1235, 0.2422)
  line L592 (0.1235, 0.2422) -> (0.1239, 0.2441)
  line L593 (0.1239, 0.2441) -> (0.1233, 0.2479)
  line L594 (0.1233, 0.2479) -> (0.1038, 0.2883)
  line L595 (0.1038, 0.2883) -> (0.1012, 0.2912)
  line L596 (0.1012, 0.2912) -> (0.0995, 0.292)
  line L597 (0.0995, 0.292) -> (0.0979, 0.2924)
  line L598 (0.0979, 0.2924) -> (0.0964, 0.2927)
  line L599 (0.0964, 0.2927) -> (0.0949, 0.2928)
  line L600 (0.0949, 0.2928) -> (0.0935, 0.2928)
  line L601 (0.0935, 0.2928) -> (0.0907, 0.2927)
  line L602 (0.0907, 0.2927) -> (0.088, 0.2923)
  line L603 (0.088, 0.2923) -> (0.0854, 0.2917)
  line L604 (0.0854, 0.2917) -> (0.0802, 0.2904)
  line L605 (0.0802, 0.2904) -> (0.0748, 0.2895)
  line L606 (0.0748, 0.2895) -> (0.0693, 0.289)
  line L607 (0.0693, 0.289) -> (0.0637, 0.2888)
  line L608 (0.0637, 0.2888) -> (0.058, 0.2889)
  line L609 (0.058, 0.2889) -> (0.0523, 0.2892)
  line L610 (0.0523, 0.2892) -> (0.0465, 0.2898)
  line L611 (0.0465, 0.2898) -> (0.0406, 0.2906)
  line L612 (0.0406, 0.2906) -> (0.0347, 0.2915)
  line L613 (0.0347, 0.2915) -> (0.0287, 0.2927)
  line L614 (0.0287, 0.2927) -> (0.0227, 0.2941)
  line L615 (0.0227, 0.2941) -> (0.0167, 0.2957)
  line L616 (0.0167, 0.2957) -> (0.0055, 0.3447)
  line L617 (0.0055, 0.3447) -> (0.0102, 0.3488)
  line L618 (0.0102, 0.3488) -> (0.015, 0.3527)
  line L619 (0.015, 0.3527) -> (0.0199, 0.3563)
  line L620 (0.0199, 0.3563) -> (0.0248, 0.3598)
  line L621 (0.0248, 0.3598) -> (0.0298, 0.363)
  line L622 (0.0298, 0.363) -> (0.0348, 0.366)
  line L623 (0.0348, 0.366) -> (0.0398, 0.3688)
  line L624 (0.0398, 0.3688) -> (0.0449, 0.3714)
  line L625 (0.0449, 0.3714) -> (0.05, 0.3736)
  line L626 (0.05, 0.3736) -> (0.0552, 0.3755)
  line L627 (0.0552, 0.3755) -> (0.0604, 0.3771)
  line L628 (0.0604, 0.3771) -> (0.0656, 0.3782)
  line L629 (0.0656, 0.3782) -> (0.0682, 0.3788)
  line L630 (0.0682, 0.3788) -> (0.0708, 0.3796)
  line L631 (0.0708, 0.3796) -> (0.0734, 0.3807)
  line L632 (0.0734, 0.3807) -> (0.0747, 0.3813)
  line L633 (0.0747, 0.3813) -> (0.076, 0.3821)
  line L634 (0.076, 0.3821) -> (0.0772, 0.383)
  line L635 (0.0772, 0.383) -> (0.0785, 0.3841)
  line L636 (0.0785, 0.3841) -> (0.0797, 0.3855)
  line L637 (0.0797, 0.3855) -> (0.0808, 0.3892)
  line L638 (0.0808, 0.3892) -> (0.0808, 0.4341)
  line L639 (0.0808, 0.4341) -> (0.0797, 0.4378)
  circle A0 centre (0.4117, 0.4117) radius 0.057
  point P0 (0, 0)
  dimension "d8" = 0.114
  constraints: 1280 end point, 253 parallel, 34 perpendicular, 1 centre point, 2 other
  measures "d8" diameter of A0
extrude "Extrusion3" add sketch "Sketch4" along normal blind 0.3 contours L0 L1 L2 L3 L4 L5 L6 L7 L8 L9 L10 L11 L12 L13 L14 L15 L16 L17 L18 L19 L20 L21 L22 L23 | L25 L27 L29 L30 L31 L32 L33 L34 L35 L36 L37 L38 L39 L40 L41 L42 L43 L44 L45 L46 L47 L48 L49 L50 L51 L52 L53 L54 L55 L56 L57 L58 L59 L61 L63 L65 L66 L67 L69 L71 L73 L75 L76 L77 L78 L79 L80 L81 L82 L83 L84 L85 L86 L87 L88 L89 L90 L91 L92 L93 L94 L95 L96 L97 L98 L99 L100 L101 L102 L103 L105 L107 L109 L110 L111 L113 L115 L117 L118 L119 L120 L121 L122 L123 L124 L125 L126 L127 L128 L129 L130 L131 L132 L133 L134 L135 L136 L137 L138 L139 L140 L141 L142 L143 L144 L145 L146 L147 L149 L151 L153 L154 L155 L157 L159 L161 L162 L163 L164 L165 L166 L167 L168 L169 L170 L171 L172 L173 L174 L175 L176 L177 L178 L179 L180 L181 L182 L183 L184 L185 L186 L187 L188 L189 L190 L191 L193 L195 L197 L198 L199 L201 L203 L205 L206 L207 L208 L209 L210 L211 L212 L213 L214 L215 L216 L217 L218 L219 L220 L221 L222 L223 L224 L225 L226 L227 L228 L229 L230 L231 L232 L233 L234 L235 L237 L239 L241 L242 L243 L245 L247 L249 L250 L251 L252 L253 L254 L255 L256 L257 L258 L259 L260 L261 L262 L263 L264 L265 L266 L267 L268 L269 L270 L271 L272 L273 L274 L275 L276 L277 L279 L281 L283 L285 L286 L287 L289 L291 L293 L294 L295 L296 L297 L298 L299 L300 L301 L302 L303 L304 L305 L306 L307 L308 L309 L310 L311 L312 L313 L314 L315 L316 L317 L318 L319 L320 L321 L322 L323 L325 L327 L329 L330 L331 L333 L335 L337 L338 L339 L340 L341 L342 L343 L344 L345 L346 L347 L348 L349 L350 L351 L352 L353 L354 L355 L356 L357 L358 L359 L360 L361 L362 L363 L364 L365 L366 L367 L369 L371 L373 L374 L375 L377 L379 L381 L383 L384 L385 L386 L387 L388 L389 L390 L391 L392 L393 L394 L395 L396 L397 L398 L399 L400 L401 L402 L403 L404 L405 L406 L407 L408 L409 L410 L411 L413 L415 L417 L418 L419 L421 L423 L425 L426 L427 L428 L429 L430 L431 L432 L433 L434 L435 L436 L437 L438 L439 L440 L441 L442 L443 L444 L445 L446 L447 L448 L449 L450 L451 L452 L453 L454 L455 L457 L459 L461 L462 L463 L465 L467 L469 L470 L471 L472 L473 L474 L475 L476 L477 L478 L479 L480 L481 L482 L483 L484 L485 L486 L487 L488 L489 L490 L491 L492 L493 L494 L495 L496 L497 L498 L499 L501 L503 L505 L506 L507 L509 L511 L513 L514 L515 L516 L517 L518 L519 L520 L521 L522 L523 L524 L525 L526 L527 L528 L529 L530 L531 L532 L533 L534 L535 L536 L537 L538 L539 L540 L541 L542 L543 L545 L547 L549 L550 L551 L554 L556 L557 L558 L559 L560 L561 L562 L563 L564 L565 L566 L567 L568 L569 L570 L571 L572 L573 L574 L575 L576 L577 L578 L579 L580 L581 L582 L583 L584 L585 L587 L589 L591 L593 L594 L595 L597 L599 L601 L602 L603 L604 L605 L606 L607 L608 L609 L610 L611 L612 L613 L614 L615 L616 L617 L618 L619 L620 L621 L622 L623 L624 L625 L626 L627 L628 L629 L630 L631 L633 L635 L637 L638 L639